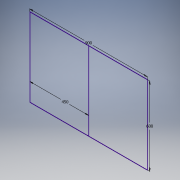
# Autodesk Inventor part: Кресло бок
Saved by Autodesk Inventor 2019 (Build 230136000, 136)
## iProperties
Created: 2018-10-09
Part Number: Кресло бок
Material: Древесина (дуб)
Document SubType Name: Modeling
Designer: Андреев Н.Л.
Density: 0.76 g/cm^3
Appearance: Белый дуб — натуральный — с умеренным глянцем
Author: Андреев Н.Л.
Autodesk Inventor part; units mm, degrees
ref_plane "YZ Plane" through (0, 0, 0) normal (1, 0, 0) x (0, 1, 0)
ref_plane "XZ Plane" through (0, 0, 0) normal (0, 1, 0) x (-1, 0, 0)
ref_plane "XY Plane" through (0, 0, 0) normal (0, 0, 1) x (1, 0, 0)
sketch "Эскиз1" plane through (0, 0, 0) normal (0, 0, 1) x (1, 0, 0)
  line L0 (0, 0) -> (900, 0) construction
  line L1 (900, 0) -> (900, 600) construction
  line L2 (900, 600) -> (0, 600) construction
  line L3 (0, 600) -> (0, 0) construction
  line L4 (450, 0) -> (450, 600) construction
  line L5 (0, 0) -> (300.7975, 83.9601) construction
  arc A0 (300.7975, 83.9601) -> (397.9046, 211.8842) centre (265.0907, 211.8842) ccw construction
  line L6 (397.9046, 211.8842) -> (397.9046, 458.8432) construction
  arc A1 (397.9046, 458.8432) -> (329.7441, 559.0793) centre (290.1213, 458.8432) ccw construction
  line L7 (329.7441, 559.0793) -> (0, 648.6149) construction
  line L8 (370.878, 131.5811) -> (952.3323, -102.4791) construction
  line L9 (647.6145, 500.9424) -> (647.6145, 136.0829) construction
  arc A2 (578.6712, 47.9354) -> (647.6145, 136.0829) centre (556.7924, 136.0829) ccw construction
  line L10 (427.9046, 458.8432) -> (427.9046, 211.8842)
  arc A3 (305.9316, 54.2758) -> (427.9046, 211.8842) centre (265.0907, 211.8842) ccw
  line L11 (305.9316, 54.2758) -> (0, -25)
  line L12 (0, 628.6149) -> (312.8054, 533.2453)
  arc A4 (367.9046, 458.8432) -> (312.8054, 533.2453) centre (290.1213, 458.8432) ccw
  line L13 (367.9046, 458.8432) -> (367.9046, 211.8842)
  arc A5 (294.639, 113.4078) -> (367.9046, 211.8842) centre (265.0907, 211.8842) ccw
  line L14 (294.639, 113.4078) -> (0, 25)
  line L15 (0, 668.6149) -> (0, 628.6149)
  line L16 (0, 25) -> (0, -25)
  arc A6 (427.9046, 458.8432) -> (321.664, 592.9674) centre (290.1213, 458.8432) ccw
  line L17 (321.664, 592.9674) -> (0, 668.6149)
  line L18 (417.1839, 153.7805) -> (962.17, -79.496)
  arc A7 (943.569, -125.8928) -> (962.17, -79.496) centre (952.3323, -102.4791) ccw
  line L19 (943.569, -125.8928) -> (371.149, 88.3528)
  line L20 (672.6145, 500.9424) -> (672.6145, 110.3343)
  arc A8 (672.6145, 500.9424) -> (622.6275, 500.1383) centre (647.6145, 500.9424) ccw
  line L21 (622.6275, 500.1383) -> (604.007, 124.227)
  arc A9 (583.3732, 82.6446) -> (604.007, 124.227) centre (546, 127.1003) ccw
  arc A10 (652.3223, 53.1316) -> (672.6145, 110.3343) centre (581.8425, 110.3343) ccw
  dimension "d0" = 900
  dimension "d1" = 600
  dimension "d2" = 450
  dimension "d3" = 60
  dimension "d4" = 40
  dimension "d5" = 50
  dimension "d6" = 80
  dimension "d7" = 25
  dimension "d8" = 40
  dimension "d9" = 25
  dimension "d10" = 75
  dimension "d11" = 70
  constraints: 44 end point, 25 point on circle, 17 tangent, 11 centre point, 7 vertical, 5 point on line, 4 concentric, 4 midpoint, 3 parallel, 2 coincident, 2 perpendicular, 2 vertical alignment, 1 collinear, 1 horizontal, 7 other
  measures "d0" distance of L2.end L1.end
  measures "d1" distance of L1.end L0.end
  measures "d2" distance between parallel lines of L3 L4
  measures "d3" distance between parallel lines of L13 L10
  measures "d4" distance of L15.start L12.start
  measures "d5" distance of L14.end L11.end
  measures "d6" distance of L18.start L19.end
  measures "d7" radius of A7
  measures "d8" distance from line of L8 L19.end
  measures "d9" radius of A8
  measures "d10" distance of A9.start A10.start
  measures "d11" distance of L21.end L20.end
extrude "Выдавливание1" add sketch "Эскиз1" along normal mid plane 22
sketch "Эскиз2" plane through (672.6145, 110.3343, 11) normal (1, 0, 0) x (0, 0, -1)
  line L0 (0, 390.6081) -> (22, 390.6081) construction
  line L1 (0, 0) -> (0, 390.6081) construction
  line L2 (22, 0) -> (0, 0) construction
  line L3 (22, 390.6081) -> (22, 0) construction
  line L4 (11, 390.6081) -> (11, 65.1808) construction
  line L5 (62.2938, 390.6081) -> (62.2938, 65.1808)
  line L6 (-40.2938, 65.1808) -> (-40.2938, 390.6081)
  arc A0 (62.2938, 390.6081) -> (-40.2938, 390.6081) centre (11, 390.6081) ccw
  arc A1 (-40.2938, 65.1808) -> (62.2938, 65.1808) centre (11, 65.1808) ccw
  point P0 (11, -110.3343)
  point P1 (11, 227.8944)
  constraints: 8 end point, 4 point on circle, 4 tangent, 2 centre point, 2 midpoint, 2 parallel
extrude "Выдавливание2" add sketch "Эскиз2" along normal blind 22
